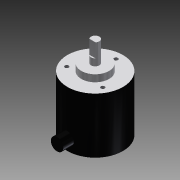
# Autodesk Inventor part: Encoder
Saved by Autodesk Inventor 2014 SP1 (Build 180222100, 222)
## iProperties
Created: 2015-03-16
Part Number: Encoder
Material: Generic
Document SubType Name: Modeling
Designer: david
Density: 1 g/cm^3
Appearance: Default
Encoder_Shaft_Diameter: 6,000 mm
Encoder_Shaft_Meplat_Depth: 1,000 mm
Encoder_Shaft_Meplat_Lenght: 10,000 mm
Encoder_Shaft_Length: 15,000 mm
Encoder_Bearing_Height: 5,000 mm
Encoder_Body_Length: 40,000 mm
Encoder_Body_Diameter: 40,000 mm
Encoder_Bearing_Diameter: 20,000 mm
Encoder_FixationHole_Size: 2,800 mm
Encoder_FixationHole_DistanceToCenter: 15,000 mm
Encoder_CableFixation_Diameter: 9,000 mm
Encoder_CableFixation_DistanceToTop: 32,000 mm
Author: david
Autodesk Inventor part; units mm, degrees
ref_plane "YZ Plane" through (0, 0, 0) normal (1, 0, 0) x (0, 1, 0)
ref_plane "XZ Plane" through (0, 0, 0) normal (0, 1, 0) x (-1, 0, 0)
sketch "BodySketch" plane through (0, 0, 0) normal (0, 1, 0) x (-1, 0, 0)
  circle A0 centre (0, 0) radius 20
  dimension "Encoder_Body_Diameter" = 40
  constraints: 1 centre point, 1 coincident
  measures "Encoder_Body_Diameter" diameter of A0
extrude "Body" add sketch "BodySketch" along normal blind 40
sketch "BearingSketch" plane through (0, 40, 0) normal (0, 1, 0) x (1, 0, 0)
  circle A0 centre (0, 0) radius 20 projected
  circle A1 centre (0, 0) radius 10
  dimension "Encoder_Bearing_Diameter" = 20
  constraints: 1 centre point, 1 coincident
  measures "Encoder_Bearing_Diameter" diameter of A1
extrude "Bearing" add sketch "BearingSketch" along normal blind 5 contours A1
sketch "ShaftSketch" plane through (0, 45, 0) normal (0, 1, 0) x (1, 0, 0)
  circle A0 centre (0, 0) radius 10 projected
  circle A1 centre (0, 0) radius 3
  dimension "d12" = 6
  constraints: 1 centre point, 1 coincident
  measures "d12" diameter of A1
extrude "Shaft" add sketch "ShaftSketch" along normal blind 15 contours A1
sketch "MeplatSketch" plane through (0, 60, 0) normal (0, 1, 0) x (1, 0, 0)
  circle A0 centre (0, 0) radius 3 projected
  line L0 (-2.2361, -2) -> (2.2361, -2)
  dimension "d16" = 1
  constraints: 2 end point, 2 point on circle, 1 horizontal
  measures "d16" distance edge to line of A0 L0
extrude "Meplat" cut sketch "MeplatSketch" against normal blind 10 contours L0 A0 picked at (-0.5653, -2.1582)
sketch "FixationHoleSketch" plane through (0, 40, 0) normal (0, 1, 0) x (1, 0, 0)
  circle A0 centre (0, 0) radius 10 projected
  circle A1 centre (0, 0) radius 20 projected
  circle A2 centre (0, 15) radius 1.4
  line L0 (0, 0) -> (0, 35.8513) construction
  circle A3 centre (-12.9904, -7.5) radius 1.4
  circle A4 centre (12.9904, -7.5) radius 1.4
  dimension "Encoder_FixationHole_Size" = 2.8
  dimension "Encoder_FixationHole_DistanceToCenter" = 15
  dimension "d23" = 360
  constraints: 3 centre point, 2 end point, 1 point on line, 1 vertical, 7 other
  measures "Encoder_FixationHole_Size" diameter of A2
  measures "Encoder_FixationHole_DistanceToCenter" distance of A0.centre A2.centre
extrude "FixationHole" cut sketch "FixationHoleSketch" against normal blind 6 contours A2 | A3 | A4
ref_plane "Work Plane1" through (0, 0, 20) normal (0, 0, 1) x (1, 0, 0)
sketch "CableFixationSketch" plane through (0, 0, 20) normal (0, 0, 1) x (1, 0, 0)
  circle A0 centre (0, 8) radius 4.5
  line L0 (0, 0) -> (0, 79.6657) construction
  dimension "Encoder_CableFixation_Diameter" = 9
  dimension "Encoder_CableFixation_DistanceToBase" = 8
  constraints: 2 end point, 1 centre point, 1 point on line, 1 vertical
  measures "Encoder_CableFixation_Diameter" diameter of A0
  measures "Encoder_CableFixation_DistanceToBase" distance of L0.start A0.centre
extrude "CableFixation" add sketch "CableFixationSketch" along normal blind 7.5
equation "\"d12\" = Encoder_Shaft_Diameter"
equation "\"d13\" = Encoder_Shaft_Length"
equation "\"d16\" = Encoder_Shaft_Meplat_Depth"
equation "\"d17\" = Encoder_Shaft_Meplat_Lenght"
equation "\"Encoder_Shaft_Diameter\" = 6"
equation "\"Encoder_Shaft_Length\" = 15"
equation "\"Encoder_Shaft_Meplat_Depth\" = 1"
equation "\"Encoder_Shaft_Meplat_Lenght\" = 10"
equation "\"Encoder_CableFixation_DistanceToTop\" = Encoder_Body_Length - Encoder_CableFixation_DistanceToBase"
equation "\"Encoder_Body_Length\" = 40"
body "Solid1"
